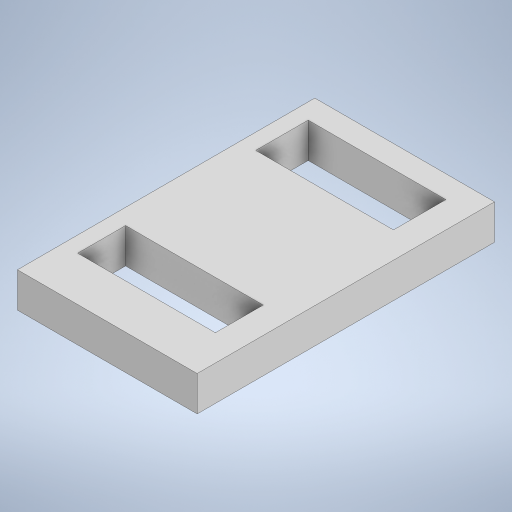
# Autodesk Inventor part: подшипник_крепеж
Saved by Autodesk Inventor 2024.2 (Build 282272000, 272)
## iProperties
Created: 2026-01-05
Part Number: подшипник_крепеж
Material: Типовые
Document SubType Name: Modeling
Designer: Service
Density: 1 g/cm^3
Appearance: По умолчанию
Author: Service
Autodesk Inventor part; units mm, degrees
ref_plane "YZ Plane" through (0, 0, 0) normal (1, 0, 0) x (0, 1, 0)
ref_plane "XZ Plane" through (0, 0, 0) normal (0, 1, 0) x (-1, 0, 0)
ref_plane "XY Plane" through (0, 0, 0) normal (0, 0, 1) x (1, 0, 0)
sketch "Эскиз1" plane through (0, 0, 0) normal (0, 1, 0) x (-1, 0, 0)
  line L0 (9.374, 18.1547) -> (1.5, 18.1547)
  line L1 (1.5, 18.1547) -> (1.5, 15.4147)
  line L2 (1.5, 15.4147) -> (9.374, 15.4147)
  line L3 (9.374, 15.4147) -> (9.374, 18.1547)
  line L4 (9.374, 7.9747) -> (1.5, 7.9747)
  line L5 (1.5, 7.9747) -> (1.5, 4.9747)
  line L6 (1.5, 4.9747) -> (9.374, 4.9747)
  line L7 (9.374, 4.9747) -> (9.374, 7.9747)
  line L8 (10.2755, 20.6947) -> (0, 20.6947)
  line L9 (0, 20.6947) -> (0, 3.6947)
  line L10 (0, 3.6947) -> (10.2755, 3.6947)
  line L11 (10.2755, 3.6947) -> (10.2755, 20.6947)
  point P0 (0, 0)
  dimension "d3" = 17
  dimension "d4" = 7.874
  dimension "d5" = 2.74
  dimension "d6" = 2.54
  dimension "d7" = 7.44
  dimension "d8" = 1.5
  dimension "d11" = 3
  constraints: 24 end point, 6 parallel, 3 horizontal, 3 perpendicular, 1 point on line
  measures "d3" distance of L8.end L9.end
  measures "d4" distance of L1.end L2.end
  measures "d5" distance of L0.end L1.end
  measures "d6" distance between parallel lines of L8 L0
  measures "d7" distance between parallel lines of L2 L4
  measures "d8" distance between parallel lines of L1 L9
  measures "d11" distance of L4.end L5.end
extrude "Выдавливание1" add sketch "Эскиз1" along normal blind 2
sketch "Эскиз3" plane through (0, 0, 0) normal (0, -1, 0) x (1, 0, 0)
  line L0 (-8.9898, 13.0238) -> (-0.8671, 13.0238) construction
  line L1 (-0.8671, 13.0238) -> (-0.8671, 9.5038) construction
  line L2 (-0.8671, 9.5038) -> (-8.9898, 9.5038) construction
  line L3 (-8.9898, 9.5038) -> (-8.9898, 13.0238) construction
  spline S0 degree 2 poles (-7.8313, 9.8672) (-8.1623, 9.8672) (-8.6267, 10.0055) (-8.8317, 10.1043) knots 0 0 0 1 2 2 2
  line L4 (-8.8317, 10.1043) -> (-8.8317, 10.6131)
  line L5 (-8.8317, 10.6131) -> (-8.802, 10.6131)
  spline S1 degree 2 poles (-8.802, 10.6131) (-8.602, 10.4254) (-8.0956, 10.2179) (-7.861, 10.2179) knots 0 0 0 1 2 2 2
  spline S2 degree 2 poles (-7.861, 10.2179) (-7.525, 10.2179) (-7.1817, 10.497) (-7.1817, 10.7267) knots 0 0 0 1 2 2 2
  spline S3 degree 2 poles (-7.1817, 10.7267) (-7.1817, 10.9095) (-7.362, 11.1367) (-7.5572, 11.1936) knots 0 0 0 1 2 2 2
  spline S4 degree 2 poles (-7.5572, 11.1936) (-7.6979, 11.2331) (-7.9326, 11.2874) (-8.108, 11.3319) knots 0 0 0 1 2 2 2
  spline S5 degree 2 poles (-8.108, 11.3319) (-8.2661, 11.3739) (-8.5155, 11.4998) (-8.6119, 11.6011) knots 0 0 0 1 2 2 2
  spline S6 degree 2 poles (-8.6119, 11.6011) (-8.7057, 11.7024) (-8.8095, 11.9741) (-8.8095, 12.1519) knots 0 0 0 1 2 2 2
  spline S7 degree 2 poles (-8.8095, 12.1519) (-8.8095, 12.5224) (-8.2315, 13.0238) (-7.7844, 13.0238) knots 0 0 0 1 2 2 2
  spline S8 degree 2 poles (-7.7844, 13.0238) (-7.5275, 13.0238) (-7.073, 12.9226) (-6.8779, 12.8262) knots 0 0 0 1 2 2 2
  line L6 (-6.8779, 12.8262) -> (-6.8779, 12.3421)
  line L7 (-6.8779, 12.3421) -> (-6.9075, 12.3421)
  spline S9 degree 2 poles (-6.9075, 12.3421) (-7.0533, 12.4755) (-7.5078, 12.6731) (-7.7572, 12.6731) knots 0 0 0 1 2 2 2
  spline S10 degree 2 poles (-7.7572, 12.6731) (-8.0388, 12.6731) (-8.3871, 12.4088) (-8.3871, 12.1939) knots 0 0 0 1 2 2 2
  spline S11 degree 2 poles (-8.3871, 12.1939) (-8.3871, 12.0012) (-8.1821, 11.7715) (-7.9894, 11.7197) knots 0 0 0 1 2 2 2
  spline S12 degree 2 poles (-7.9894, 11.7197) (-7.861, 11.6851) (-7.488, 11.5962) (-7.3645, 11.5591) knots 0 0 0 1 2 2 2
  spline S13 degree 2 poles (-7.3645, 11.5591) (-7.0508, 11.4628) (-6.7593, 11.075) (-6.7593, 10.7909) knots 0 0 0 1 2 2 2
  spline S14 degree 2 poles (-6.7593, 10.7909) (-6.7593, 10.6106) (-6.9051, 10.2648) (-7.036, 10.1438) knots 0 0 0 1 2 2 2
  spline S15 degree 2 poles (-7.036, 10.1438) (-7.1817, 10.0104) (-7.5522, 9.8672) (-7.8313, 9.8672) knots 0 0 0 1 2 2 2
  line L8 (-4.1362, 12.9695) -> (-5.1859, 9.9215)
  line L9 (-5.1859, 9.9215) -> (-5.6231, 9.9215)
  line L10 (-5.6231, 9.9215) -> (-6.6729, 12.9695)
  line L11 (-6.6729, 12.9695) -> (-6.2382, 12.9695)
  line L12 (-6.2382, 12.9695) -> (-5.3934, 10.4377)
  line L13 (-5.3934, 10.4377) -> (-4.5487, 12.9695)
  line L14 (-4.5487, 12.9695) -> (-4.1362, 12.9695)
  spline S16 degree 2 poles (-2.5677, 9.8622) (-2.8913, 9.8622) (-3.4273, 10.0598) (-3.62, 10.2599) knots 0 0 0 1 2 2 2
  spline S17 degree 2 poles (-3.62, 10.2599) (-3.8126, 10.4624) (-4.0176, 11.0602) (-4.0176, 11.448) knots 0 0 0 1 2 2 2
  spline S18 degree 2 poles (-4.0176, 11.448) (-4.0176, 11.816) (-3.8101, 12.3989) (-3.6175, 12.6064) knots 0 0 0 1 2 2 2
  spline S19 degree 2 poles (-3.6175, 12.6064) (-3.4322, 12.8065) (-2.8888, 13.0238) (-2.5653, 13.0238) knots 0 0 0 1 2 2 2
  spline S20 degree 2 poles (-2.5653, 13.0238) (-2.4096, 13.0238) (-2.1281, 12.9794) (-1.9996, 12.9399) knots 0 0 0 1 2 2 2
  spline S21 degree 2 poles (-1.9996, 12.9399) (-1.8959, 12.9102) (-1.6439, 12.8015) (-1.5674, 12.762) knots 0 0 0 1 2 2 2
  line L15 (-1.5674, 12.762) -> (-1.5674, 12.2729)
  line L16 (-1.5674, 12.2729) -> (-1.6019, 12.2729)
  spline S22 degree 2 poles (-1.6019, 12.2729) (-1.6785, 12.3396) (-1.8391, 12.4607) (-1.9873, 12.5298) knots 0 0 0 1 2 2 2
  spline S23 degree 2 poles (-1.9873, 12.5298) (-2.1108, 12.5916) (-2.4294, 12.6731) (-2.6122, 12.6731) knots 0 0 0 1 2 2 2
  spline S24 degree 2 poles (-2.6122, 12.6731) (-3.0518, 12.6731) (-3.5953, 12.0111) (-3.5953, 11.4603) knots 0 0 0 1 2 2 2
  spline S25 degree 2 poles (-3.5953, 11.4603) (-3.5953, 11.154) (-3.452, 10.6946) (-3.3161, 10.5365) knots 0 0 0 1 2 2 2
  spline S26 degree 2 poles (-3.3161, 10.5365) (-3.1852, 10.3784) (-2.8147, 10.213) (-2.5825, 10.213) knots 0 0 0 1 2 2 2
  spline S27 degree 2 poles (-2.5825, 10.213) (-2.4121, 10.213) (-2.0713, 10.2624) (-1.9552, 10.3118) knots 0 0 0 1 2 2 2
  line L17 (-1.9552, 10.3118) -> (-1.9552, 11.0997)
  line L18 (-1.9552, 11.0997) -> (-2.6616, 11.0997)
  line L19 (-2.6616, 11.0997) -> (-2.6616, 11.4554)
  line L20 (-2.6616, 11.4554) -> (-1.555, 11.4554)
  line L21 (-1.555, 11.4554) -> (-1.555, 10.124)
  spline S28 degree 2 poles (-1.555, 10.124) (-1.6316, 10.0895) (-1.8934, 9.9832) (-2.0046, 9.9511) knots 0 0 0 1 2 2 2
  spline S29 degree 2 poles (-2.0046, 9.9511) (-2.1552, 9.9067) (-2.3973, 9.8622) (-2.5677, 9.8622) knots 0 0 0 1 2 2 2
  point P0 (0, 0)
  constraints: 2 other
extrude "Выдавливание2" cut sketch "Эскиз3" against normal blind 0.4
